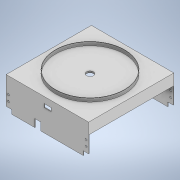
# Autodesk Inventor part: Upper_Housing
Saved by Autodesk Inventor 2022 (Build 260153000, 153)
## iProperties
Created: 2022-03-18
Part Number: Upper_Housing
Material: Generic
Document SubType Name: Modeling
Designer: Hajar
Density: 1 g/cm^3
Appearance: Default
Author: Hajar
Autodesk Inventor part; units mm, degrees
ref_plane "YZ Plane" through (0, 0, 0) normal (1, 0, 0) x (0, 1, 0)
ref_plane "XZ Plane" through (0, 0, 0) normal (0, 1, 0) x (-1, 0, 0)
ref_plane "XY Plane" through (0, 0, 0) normal (0, 0, 1) x (1, 0, 0)
sketch "Sketch2" plane through (0, 0, 0) normal (0, 0, 1) x (1, 0, 0)
  line L0 (59.5, -20) -> (-59.5, -20)
  line L1 (-59.5, -20) -> (-59.5, 20)
  line L2 (-59.5, 20) -> (59.5, 20)
  line L3 (59.5, 20) -> (59.5, -20)
  line L4 (59.5, -20) -> (-59.5, 20) construction
  line L5 (-59.5, -20) -> (59.5, 20) construction
  line L6 (-59.5, -20) -> (-51.5, -20) construction
  line L7 (-51.5, -20) -> (-51.5, 4) construction
  line L8 (-51.5, 4) -> (-59.5, 4) construction
  line L9 (-59.5, 4) -> (-59.5, -20) construction
  circle A0 centre (-56.714, -3.7) radius 1.4
  circle A1 centre (-56.714, -12.2) radius 1.4
  line L10 (59.5, -20) -> (51.5, -20) construction
  line L11 (51.5, -20) -> (51.5, 4) construction
  line L12 (51.5, 4) -> (59.5, 4) construction
  line L13 (59.5, 4) -> (59.5, -20) construction
  circle A2 centre (56.4, -3.7) radius 1.4
  circle A3 centre (56.4, -12.2) radius 1.4
  line L14 (-4.7439, 11) -> (5.5561, 11)
  line L15 (5.5561, 11) -> (5.5561, 6)
  line L16 (5.5561, 6) -> (-4.7439, 6)
  line L17 (-4.7439, 6) -> (-4.7439, 11)
  line L18 (-56.714, -3.7) -> (-58.95, -3.7) construction
  point P0 (0, 0)
  dimension "d0" = 119
  dimension "d1" = 40
  dimension "d2" = 8
  dimension "d3" = 24
  dimension "d4" = 2.8
  dimension "d5" = 7.7
  dimension "d6" = 5.214
  dimension "d7" = 2.8
  dimension "d8" = 8.5
  dimension "d9" = 8
  dimension "d10" = 24
  dimension "d12" = 2.8
  dimension "d13" = 7.7
  dimension "d15" = 4.9
  dimension "d16" = 2.8
  dimension "d17" = 8.5
  dimension "d18" = 10.3
  dimension "d19" = 5
  dimension "d20" = 26
  constraints: 38 end point, 8 parallel, 5 horizontal, 4 centre point, 4 perpendicular, 2 midpoint
  measures "d0" distance of L1.end L2.end
  measures "d1" distance of L0.end L1.end
  measures "d2" distance of L8.end L7.end
  measures "d3" distance of L7.end L6.end
  measures "d4" diameter of A0
  measures "d5" distance from line of L8 L18.start
  measures "d6" distance from line of L7 L18.start
  measures "d7" diameter of A1
  measures "d8" distance of A1.centre L18.start
  measures "d9" distance of L11.end L12.end
  measures "d10" distance of L10.end L11.end
  measures "d12" diameter of A2
  measures "d13" distance from line of L12 A2.centre
  measures "d15" distance from line of L11 A2.centre
  measures "d16" diameter of A3
  measures "d17" distance of A3.centre A2.centre
  measures "d18" distance of L15.end L16.end
  measures "d19" distance of L14.end L15.end
  measures "d20" distance between parallel lines of L0 L16
sketch "Sketch3" plane through (0, 0, 0) normal (0, 1, 0) x (-1, 0, 0)
  line L0 (-59, -61) -> (59, -61)
  line L1 (59, -61) -> (59, 61)
  line L2 (59, 61) -> (-59, 61)
  line L3 (-59, 61) -> (-59, -61)
  line L4 (-59, -61) -> (59, 61) construction
  line L5 (59, -61) -> (-59, 61) construction
  line L6 (-60, -62) -> (60, -62)
  line L7 (60, -62) -> (60, 62)
  line L8 (60, 62) -> (-60, 62)
  line L9 (-60, 62) -> (-60, -62)
  line L10 (-60, -62) -> (60, 62) construction
  line L11 (60, -62) -> (-60, 62) construction
  point P0 (0, 0)
  dimension "d21" = 118
  dimension "d22" = 122
  dimension "d23" = 120
  dimension "d24" = 124
  constraints: 24 end point, 4 midpoint, 4 parallel, 2 horizontal, 2 perpendicular
  measures "d21" distance of L2.end L1.end
  measures "d22" distance of L1.end L0.end
  measures "d23" distance of L8.end L7.end
  measures "d24" distance of L7.end L6.end
extrude "Extrusion1" add sketch "Sketch3" along normal blind 20 and the other way blind 26 contours L3 L2 L1 L0 | L9 L8 L7 L6
extrude "Extrusion2" cut sketch "Sketch2" along normal mid plane 168.5875 contours A0 | A1 | A2 | A3 | L14 L15 L16 L17
extrude "Extrusion3" cut sketch "Sketch3" along normal blind 3.83 and the other way blind 27.3 contours L3 L2 L1 L0
sketch "Sketch4" plane through (0, 20, 0) normal (0, 1, 0) x (1, 0, 0)
  circle A0 centre (0, 0) radius 50
  circle A1 centre (0, 0) radius 50.5
  circle A2 centre (0, 0) radius 5
  dimension "d33" = 100
  dimension "d34" = 101
  dimension "d35" = 10
  constraints: 3 centre point, 3 coincident
  measures "d33" diameter of A0
  measures "d34" diameter of A1
  measures "d35" diameter of A2
extrude "Extrusion4" cut sketch "Sketch4" along normal mid plane 10 contours A2
extrude "Extrusion5" add sketch "Sketch4" along normal blind 5 contours A1
sketch "Sketch5" plane through (-60, 20, 62) normal (0, 0, 1) x (1, 0, 0)
  line L0 (1, -46) -> (119, -46) projected
  line L1 (41.608, -46) -> (50.608, -46)
  line L2 (50.608, -46) -> (50.608, -34.6)
  line L3 (50.608, -34.6) -> (41.608, -34.6)
  line L4 (41.608, -34.6) -> (41.608, -46)
  point P0 (60, -20)
  dimension "d40" = 9
  dimension "d41" = 11.4
  constraints: 8 end point, 2 parallel, 1 horizontal, 1 perpendicular, 1 point on line
  measures "d40" distance of L3.end L2.end
  measures "d41" distance of L2.end L1.end
extrude "Extrusion6" cut sketch "Sketch5" against normal blind 5
sketch "Sketch6" plane through (60, -26, -62) normal (1, 0, 0) x (0, 0, -1)
  line L0 (-123, 0) -> (-123, 29.83) projected
  line L1 (-1, 0) -> (-1, 29.83) projected
  line L2 (-123, 29.83) -> (-1, 29.83)
  line L3 (-1, 29.83) -> (-1, 0)
  line L4 (-1, 0) -> (-123, 0)
  line L5 (-123, 0) -> (-123, 29.83)
  point P0 (-62, 26)
  point P1 (-124, 46)
  constraints: 8 end point, 2 parallel, 1 horizontal, 1 perpendicular
extrude "Extrusion7" cut sketch "Sketch6" along normal blind 100 and the other way blind 1000
sketch "Sketch7" plane through (-60, 20, 62) normal (0, 0, 1) x (1, 0, 0)
  line L0 (0, 0) -> (0, -46) construction
  line L1 (0, 0) -> (0, -40) construction
  line L2 (0, -46) -> (0, -16.17) construction
  line L3 (0, -40) -> (8, -40) construction
  line L4 (120, -46) -> (120, 0) construction
  line L5 (120, 0) -> (120, -40) construction
  line L6 (120, -40) -> (112, -40) construction
  line L7 (112, -40) -> (112, -46) construction
  line L8 (8, -40) -> (8, -46) construction
  line L9 (0, -46) -> (120, -46) construction
  line L10 (0, -40) -> (8, -40)
  line L11 (8, -40) -> (8, -46)
  line L12 (120, -40) -> (112, -40)
  line L13 (112, -46) -> (112, -40)
  line L14 (0, -40) -> (0, -46)
  line L15 (0, -46) -> (8, -46)
  line L16 (120, -16.17) -> (120, -46) projected
  line L17 (120, -40) -> (120, -46)
  line L18 (120, -46) -> (112, -46)
  point P0 (60, -20)
  dimension "d55" = 40
  dimension "d56" = 8
  dimension "d57" = 40
  dimension "d58" = 8
  constraints: 28 end point, 7 collinear, 4 perpendicular, 3 point on line, 1 vertical
  measures "d55" distance of L0.start L1.end
  measures "d56" distance of L1.end L3.end
  measures "d57" distance of L4.end L5.end
  measures "d58" distance of L5.end L6.end
extrude "Extrusion8" cut sketch "Sketch7" against normal blind 131.125
extrude "Extrusion9" cut sketch "Sketch3" along normal blind 17.775 contours L3 L2 L1 L0
body "Solid1"
